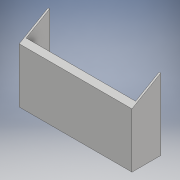
# Autodesk Inventor part: Chassi_Top_Rear
Saved by Autodesk Inventor 2018.2 (Build 222227000, 227)
## iProperties
Created: 2018-08-12
Part Number: Chassi_Top_Rear
Material: Generic
Document SubType Name: Modeling
Designer: mateu
Density: 1 g/cm^3
Appearance: Default
Author: mateu
Autodesk Inventor part; units mm, degrees
ref_plane "YZ Plane" through (0, 0, 0) normal (1, 0, 0) x (0, 1, 0)
ref_plane "XZ Plane" through (0, 0, 0) normal (0, 1, 0) x (-1, 0, 0)
ref_plane "XY Plane" through (0, 0, 0) normal (0, 0, 1) x (1, 0, 0)
sketch "Sketch1" plane through (0, 0, 0) normal (0, 0, 1) x (1, 0, 0)
  line L0 (0, 0) -> (0, -40.9)
  line L1 (0, 0) -> (160, 0)
  line L2 (160, 0) -> (160, -40.9)
  line L3 (160, -40.9) -> (157.6, -40.9)
  line L4 (157.6, -40.9) -> (157.6, -2.4)
  line L5 (157.6, -2.4) -> (2.4, -2.4)
  line L6 (2.4, -2.4) -> (2.4, -40.9)
  line L7 (2.4, -40.9) -> (0, -40.9)
  line L8 (160, -21.65) -> (157.6, -21.65)
  line L9 (2.4, -21.65) -> (0, -21.65)
  dimension "d0" = 40.9
  dimension "d1" = 160
  dimension "d2" = 2.4
  dimension "d3" = 38.5
  dimension "d4" = 155.2
  constraints: 20 end point, 4 perpendicular, 4 point on line, 2 midpoint, 2 parallel, 1 horizontal, 1 vertical
  measures "d0" distance of L0.start L0.end
  measures "d1" distance of L0.start L1.end
  measures "d2" distance of L2.end L3.end
  measures "d3" distance of L3.end L4.end
  measures "d4" distance of L4.end L5.end
extrude "Extrusion5" add sketch "Sketch1" along normal blind 77.7 contours L9 L6 L7 L0 | L2 L3 L4 L8
extrude "Extrusion6" add sketch "Sketch1" along normal blind 10 contours L1 L2 L8 L4 L5 L6 L9 L0
sketch "Sketch6" plane through (160, -40.9, 77.7) normal (1, 0, 0) x (0, 0, -1)
  line L0 (0, 0) -> (0, 19.25) projected
  line L1 (0, 19.25) -> (0, 0)
  line L2 (77.7, 0) -> (0, 0) projected
  line L3 (0, 0) -> (-11.114, 19.25)
  line L4 (0, 0) -> (22.228, 0) construction
  line L5 (-11.114, 19.25) -> (0, 19.25)
  point P0 (77.7, 40.9)
  dimension "d21" = 120
  constraints: 8 end point, 1 collinear, 1 equal length, 1 horizontal, 1 parallel
  measures "d21" angle of L4 L3
extrude "Extrusion7" add sketch "Sketch6" against normal blind 2.4
sketch "Sketch7" plane through (0, -40.9, 77.7) normal (-1, 0, 0) x (0, 0, 1)
  line L0 (0, 0) -> (0, 19.25) projected
  line L1 (0, 19.25) -> (0, 0)
  line L2 (-67.7, 19.25) -> (11.114, 19.25) projected
  line L3 (0, 0) -> (11.114, 19.25)
  line L4 (11.114, 19.25) -> (0, 19.25)
  point P0 (-77.7, 40.9)
  constraints: 6 end point, 1 collinear, 1 vertical
extrude "Extrusion8" add sketch "Sketch7" against normal blind 2.4
sketch "Sketch8" plane through (2.4, -40.9, 0) normal (1, 0, 0) x (0, 0, -1)
  line L0 (0, 0) -> (0, 2.4)
  line L1 (0, 0) -> (0, 38.5) projected
  line L2 (0, 2.4) -> (-79.0856, 2.4)
  line L3 (-88.814, 19.25) -> (-77.7, 0) projected
  line L4 (-77.7, 0) -> (0, 0)
  point P0 (0, 40.9)
  dimension "d26" = 2.4
  constraints: 6 end point, 2 perpendicular, 2 point on line
  measures "d26" distance of L0.start L0.end
extrude "Extrusion9" add sketch "Sketch8" along normal blind 157
sketch "Sketch9" plane through (2.4, -21.65, 10) normal (1, 0, 0) x (0, 0, -1)
  line L0 (10, -16.85) -> (10, 19.25) projected
  line L1 (10, -16.85) -> (10, -10.85)
  line L2 (10, -10.85) -> (7.6, -10.85)
  line L3 (7.6, -10.85) -> (7.6, -16.85)
  line L4 (-69.0856, -16.85) -> (10, -16.85) projected
  line L5 (7.6, -16.85) -> (10, -16.85)
  line L6 (-69.0856, -16.85) -> (-66.6856, -16.85)
  line L7 (-66.6856, -16.85) -> (-69.6856, -11.6538)
  line L8 (-69.6856, -11.6538) -> (-72.0856, -11.6538)
  line L9 (-67.7, -19.25) -> (-78.814, 0) projected
  line L10 (-72.0856, -11.6538) -> (-69.0856, -16.85)
  point P0 (10, 21.65)
  dimension "d29" = 6
  dimension "d30" = 2.4
  dimension "d31" = 6
  dimension "d32" = 90
  dimension "d33" = 2.4
  dimension "d34" = 6
  dimension "d35" = 60
  dimension "d36" = 120
  constraints: 16 end point, 3 point on line, 2 perpendicular, 1 collinear
  measures "d29" distance of L0.start L1.end
  measures "d30" distance of L1.end L2.end
  measures "d31" distance of L2.end L3.end
  measures "d32" angle of L3 L2
  measures "d33" distance of L4.start L6.end
  measures "d34" distance of L6.end L7.end
  measures "d35" angle of L7 L6
  measures "d36" angle of L8 L7
extrude "Extrusion10" add sketch "Sketch9" along normal blind 157
sketch "Sketch10" plane through (0, -40.9, 0) normal (-1, 0, 0) x (0, 0, 1)
  line L0 (10, 40.9) -> (10, 19.25)
  line L1 (10, 19.25) -> (88.814, 19.25)
  line L2 (10, 19.25) -> (88.814, 19.25) projected
  line L3 (88.814, 19.25) -> (101.3136, 40.9)
  line L4 (88.814, 19.25) -> (113.8133, 19.25) construction
  line L5 (101.3136, 40.9) -> (10, 40.9)
  point P0 (0, 40.9)
  dimension "d39" = 60
  constraints: 10 end point, 2 horizontal, 1 equal length, 1 perpendicular, 1 vertical
  measures "d39" angle of L4 L3
extrude "Extrusion11" add sketch "Sketch10" against normal blind 2.4
sketch "Sketch11" plane through (160, -40.9, 0) normal (1, 0, 0) x (0, 0, -1)
  line L0 (-10, 40.9) -> (-10, 38.5) projected
  line L1 (-10, 40.9) -> (-10, 19.25)
  line L2 (-10, 19.25) -> (-88.814, 19.25) projected
  line L3 (-10, 19.25) -> (-88.814, 19.25)
  line L4 (-88.814, 19.25) -> (-101.3136, 40.9)
  line L5 (-101.3136, 40.9) -> (-10, 40.9)
  point P0 (0, 40.9)
  constraints: 8 end point, 1 parallel, 1 perpendicular, 1 vertical
extrude "Extrusion12" add sketch "Sketch11" against normal blind 2.4
body "Solid2"
